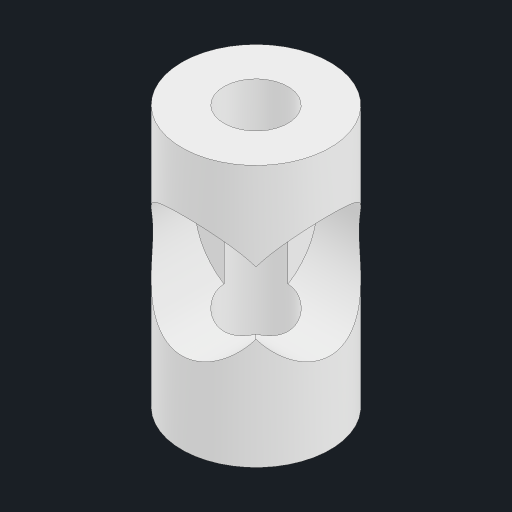
# Autodesk Inventor part: motor_shaft_adapter
Saved by Autodesk Inventor 2023 (Build 270158000, 158)
## iProperties
Created: 2024-04-12
Part Number: motor_shaft_adapter
Material: ABS Plastic
Document SubType Name: Modeling
Designer: szymo
Density: 1.06 g/cm^3
Appearance: Smooth - White
Author: szymo
Autodesk Inventor part; units mm, degrees
ref_plane "YZ Plane" through (0, 0, 0) normal (1, 0, 0) x (0, 1, 0)
ref_plane "XZ Plane" through (0, 0, 0) normal (0, 1, 0) x (-1, 0, 0)
ref_plane "XY Plane" through (0, 0, 0) normal (0, 0, 1) x (1, 0, 0)
sketch "Sketch1" plane through (0, 0, 0) normal (0, 1, 0) x (-1, 0, 0)
  circle A0 centre (0, 0) radius 1.1
  circle A1 centre (0, 0) radius 2.55
  dimension "d0" = 2.2
  dimension "d1" = 5.1
  constraints: 2 centre point, 2 coincident
  measures "d0" diameter of A0
  measures "d1" diameter of A1
extrude "Extrusion1" add sketch "Sketch1" along normal blind 9
sketch "Sketch2" plane through (0, 0, 0) normal (0, 0, 1) x (1, 0, 0)
  line L0 (2.55, 9) -> (-2.55, 9) projected
  line L1 (2.55, 0) -> (-2.55, 0) projected
  line L2 (-2.55, 0) -> (-2.55, 9) projected
  line L3 (-2.55, 7) -> (2.5173, 7)
  line L4 (2.55, 9) -> (-2.55, 9) projected
  line L5 (0, 9) -> (0, 0)
  circle A0 centre (0, 4.9) radius 2.1
  dimension "d4" = 2
  dimension "d5" = 4.2
  constraints: 4 end point, 2 point on line, 1 centre point, 1 horizontal, 1 midpoint, 1 parallel, 1 tangent, 1 vertical
  measures "d4" distance between parallel lines of L0 L3
  measures "d5" diameter of A0
extrude "Extrusion2" cut sketch "Sketch2" along normal blind 12 contours A0 L5 | L5 A0
sketch "Sketch3" plane through (0, 0, 0) normal (1, 0, 0) x (0, 1, 0)
  line L0 (9, -2.55) -> (9, 2.55) projected
  line L1 (0, -2.55) -> (0, 2.55) projected
  line L2 (0, 2.55) -> (9, 2.55) projected
  line L3 (7, 2.55) -> (7, -2.525)
  line L4 (9, 1.1) -> (9, -1.1) projected
  line L5 (9, 0) -> (0, 0)
  circle A0 centre (4.9, 0) radius 2.1
  point P0 (4.9, 1.4465)
  dimension "d8" = 2
  dimension "d9" = 4.2
  constraints: 4 end point, 2 point on line, 1 centre point, 1 horizontal, 1 midpoint, 1 parallel, 1 perpendicular, 1 tangent
  measures "d8" distance between parallel lines of L0 L3
  measures "d9" diameter of A0
extrude "Extrusion3" cut sketch "Sketch3" along normal up to next contours A0 L5 | L5 A0
body "Solid1"
